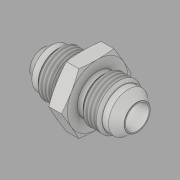
# Autodesk Inventor part: AN815-8D
Saved by Autodesk Inventor 2019 (Build 230136000, 136)
## iProperties
Created: 2018-11-23
Part Number: AN815-8D
Material: Aluminum 2014-T6
Document SubType Name: Modeling
Designer: erics
Density: 2.78927 g/cm^3
Appearance: Satin
Mass: 23.5586 g
Surface Area: 44.2792 cm^2
Volume: 8.44616 cm^3
Author: erics
Autodesk Inventor part; units mm, degrees
ref_plane "YZ Plane" through (0, 0, 0) normal (1, 0, 0) x (0, 1, 0)
ref_plane "XZ Plane" through (0, 0, 0) normal (0, 1, 0) x (-1, 0, 0)
ref_plane "XY Plane" through (0, 0, 0) normal (0, 0, 1) x (1, 0, 0)
sketch "Sketch4" plane through (0, 0, 0) normal (0, 0, 1) x (1, 0, 0)
  line L0 (0, 0) -> (0, 5.4102)
  line L1 (0.0506, 5.5116) -> (3.7586, 8.3058)
  line L2 (3.7586, 8.3058) -> (6.321, 8.3058)
  line L3 (6.5006, 8.3802) -> (7.6454, 9.525)
  line L4 (7.6454, 9.525) -> (13.1572, 9.525)
  line L5 (13.1572, 9.525) -> (14.2258, 8.4564)
  line L6 (14.4054, 8.382) -> (16.6878, 8.382)
  line L7 (16.6878, 8.382) -> (16.6878, 0)
  line L8 (16.6878, 0) -> (0, 0)
  arc A0 (0.0506, 5.5116) -> (0, 5.4102) centre (0.127, 5.4102) ccw
  arc A1 (6.321, 8.3058) -> (6.5006, 8.3802) centre (6.321, 8.5598) ccw
  arc A2 (14.2258, 8.4564) -> (14.4054, 8.382) centre (14.4054, 8.636) ccw
  point P0 (6.4262, 8.3058)
  point P1 (14.3002, 8.382)
  dimension "d26" = 45
  dimension "d28" = 16.6878
  dimension "d29" = 0.127
  dimension "d30" = 5.4102
  dimension "d31" = 37
  dimension "d32" = 6.4262
  dimension "d33" = 8.3058
  dimension "d34" = 0.254
  dimension "d35" = 8.382
  dimension "d36" = 9.525
  dimension "d37" = 45
  dimension "d39" = 2.3876
  constraints: 18 end point, 6 point on circle, 6 tangent, 4 point on line, 3 centre point, 3 perpendicular, 1 equal radius, 1 parallel, 1 vertical
  measures "d26" angle of L4 L3
  measures "d28" distance between parallel lines of L7 L0
  measures "d29" radius of A0
  measures "d30" distance of L0.start L0.end
  measures "d31" angle of L2 L1
  measures "d32" distance from line of L0 point (6.426, 8.306)
  measures "d33" distance between parallel lines of L8 L2
  measures "d34" radius of A1
  measures "d35" distance of L6.end L7.end
  measures "d36" distance between parallel lines of L8 L4
  measures "d37" angle of L4 L5
  measures "d39" distance from line of L7 point (14.3, 8.382)
revolve "Revolution3" add sketch "Sketch4" angle 360 about axis through (16.6878, 0, 0) along (-1, 0, 0)
ref_plane "Work Plane3" through (19.8438, 0, 0) normal (-1, 0, 0) x (0, 0, 1)
sketch "Sketch5" plane through (16.6878, 8.382, 0) normal (-1, 0, 0) x (0, -1, 0)
  line L0 (-4.318, 7.3323) -> (8.382, 14.6647)
  line L1 (8.382, 14.6647) -> (21.082, 7.3323)
  line L2 (21.082, 7.3323) -> (21.082, -7.3323)
  line L3 (21.082, -7.3323) -> (8.382, -14.6647)
  line L4 (8.382, -14.6647) -> (-4.318, -7.3323)
  line L5 (-4.318, -7.3323) -> (-4.318, 7.3323)
  circle A0 centre (8.382, 0) radius 14.6647 construction
  dimension "d42" = 29.3294
  dimension "d41" = 25.4
  constraints: 12 end point, 2 coincident, 1 vertical, 16 other
  measures "d41" distance between parallel lines of L2 L5
extrude "Extrusion2" add sketch "Sketch5" against normal up to surface (3.1559 mm away)
sketch "Sketch7" plane through (0, 0, 0) normal (-1, 0, 0) x (0, 0, 1)
  circle A0 centre (0, 0) radius 5.4102 projected
  constraints: 1 coincident
hole "Hole1" at (0, 0, 0) direction (1, 0, 0) diameter 9.9314 depth 16.6878 tip angle 118 start extended yes
thread "Thread3" size "3/4-16 UNF" class "3A" standard "ANSI Unified Screw Threads" full length
sketch "Sketch8" plane through (0, 0, 0) normal (0, 1, 0) x (-1, 0, 0)
  line L0 (-14.4054, 8.382) -> (-16.6878, 8.382) construction
  line L1 (-16.6878, 7.3323) -> (-16.6878, 14.6647) construction
  line L2 (-16.6878, 7.3323) -> (-16.6878, 14.6647) construction
  line L3 (-16.6878, 14.6647) -> (-19.8438, 14.6647) construction
  line L4 (-16.6878, 7.3323) -> (-19.8437, 7.3323) construction
  line L5 (-17.2142, 14.6647) -> (-16.6878, 12.7)
  line L6 (-17.2142, 14.6647) -> (-16.6878, 14.6647)
  line L7 (-16.6878, 12.7) -> (-16.6878, 14.6647)
  line L8 (-18.2658, 14.6647) -> (-18.2658, 7.3323)
  line L9 (-16.6878, 7.3323) -> (-19.8437, 7.3323) projected
  line L10 (-19.3173, 14.6647) -> (-19.8438, 12.7)
  line L11 (-19.3173, 14.6647) -> (-19.8438, 14.6647)
  line L12 (-19.8438, 12.7) -> (-19.8438, 14.6647)
  line L13 (7.7788, 0) -> (-46.6725, 0) projected
  line L14 (-19.8437, 7.3323) -> (-19.8438, 14.6647) projected
  point P0 (0, 0)
  point P1 (-24.2189, 7.3323)
  dimension "d62" = 12.7
  dimension "d64" = 15
  constraints: 14 end point, 4 symmetric about line, 2 midpoint, 2 point on line, 1 collinear, 1 perpendicular
  measures "d62" vertical distance of L5.end point (0, 0)
  measures "d64" angle of L1 L5
revolve "Revolution5" cut sketch "Sketch8" angle 360 about axis through (-10, 0, 0) along (1, 0, 0) contours L6 L7 L5
mirror "Mirror1" about plane through (19.8438, 0, 0) normal (1, 0, 0) of "Revolution3", "Extrusion2", "Hole1", "Revolution5"
equation "\"d28\" = MS33656_J"
equation "\"d30\" = 0.5 * MS33656_D"
equation "\"d32\" = MS33656_B"
equation "\"d33\" = 0.5 * MS33656_C"
equation "\"d35\" = 0.5 * MS33656_F"
equation "\"d36\" = 0.5 * AN815_T"
equation "\"d39\" = MS33656_Q"
equation "\"d41\" = AN815_E"
equation "\"d53\" = MS33656_A"
equation "\"d62\" = 0.5 * AN815_E"
equation "\"AN815_T\" = 19.05"
equation "\"AN815_E\" = 25.4"
equation "\"AN815_M\" = 39.6875"
equation "\"MS33656_A\" = 9.9314"
equation "\"MS33656_D\" = 10.8204"
equation "\"MS33656_B\" = 6.4262"
equation "\"MS33656_C\" = 16.6116"
equation "\"MS33656_F\" = 16.764"
equation "\"MS33656_J\" = 16.6878"
equation "\"MS33656_Q\" = 2.3876"
equation "\"d79\" = -0.5 * AN815_M"
equation "\"Tube_OD\" = 12.7"
body "Solid2"
